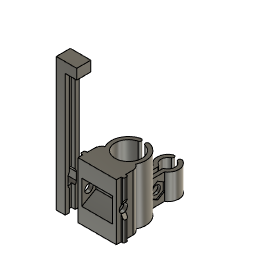
clip (Autodesk Fusion 360 design; units mm, degrees)
Autodesk Fusion 360 part; units mm, degrees
sketch "Sketch1" plane through (0, 0, 0) normal (0, 0, 1) x (1, 0, 0)
  circle A0 centre (0, 0) radius 5.25
  circle A1 centre (0, 0) radius 6.75
  line L0 (0, 1.75) -> (0, 22.5) construction
  line L1 (-7.5, -6.75) -> (7.5, -6.75)
  line L2 (2.25, 11.864) -> (2.25, 6.364)
  line L3 (-2.25, 11.864) -> (-2.25, 6.364)
  circle A2 centre (0, 15.4695) radius 2.75
  circle A3 centre (0, 15.4695) radius 4.25
  line L4 (0.75, 5.1962) -> (0.75, 19.6528)
  line L5 (-0.75, 5.1962) -> (-0.75, 19.6528)
  line L6 (-2, -4.8541) -> (-2, -2)
  arc A4 (2, -2) -> (-2, -2) centre (0, -2) ccw
  line L7 (2, -2) -> (2, -4.8541)
  line L8 (-12.5, -6.75) -> (-12.5, -8.375)
  line L9 (-12.5, -8.375) -> (-14, -8.375)
  line L10 (-14, -8.375) -> (-14, -10.625)
  line L11 (-14, -10.625) -> (-12.5, -10.625)
  line L12 (-12.5, -10.625) -> (-12.5, -12.25)
  line L13 (-16, -12.25) -> (-16, -6.75)
  line L14 (0, -9.5) -> (-16, -9.5) construction
  line L15 (-16, -6.75) -> (-12.5, -6.75)
  line L16 (-16, -12.25) -> (-12.5, -12.25)
  line L17 (-7.5, -6.75) -> (-7.5, -8.625)
  line L18 (-7.5, -8.625) -> (-8.5, -8.625)
  line L19 (-8.5, -8.625) -> (-8.5, -10.375)
  line L20 (-8.5, -10.375) -> (-7.5, -10.375)
  line L21 (-7.5, -10.375) -> (-7.5, -12.25)
  line L22 (-4, -12.25) -> (-4, -6.75)
  line L23 (-7.5, -12.25) -> (7.5, -12.25)
  line L24 (7.5, -12.25) -> (7.5, -10.375)
  line L25 (7.5, -10.375) -> (8.5, -10.375)
  line L26 (8.5, -10.375) -> (8.5, -8.625)
  line L27 (8.5, -8.625) -> (7.5, -8.625)
  line L28 (7.5, -8.625) -> (7.5, -6.75)
  line L29 (4, -6.75) -> (4, -12.25)
  line L30 (-7.5, -6.75) -> (-7.5, -5.75)
  arc A5 (-5.9559, -3.1765) -> (-7.5, -5.75) centre (-4.5833, -5.75) ccw
  line L31 (-4.5833, -5.75) -> (-5.9559, -3.1765) construction
  line L32 (7.5, -6.75) -> (7.5, -5.75)
  arc A6 (7.5, -5.75) -> (5.9559, -3.1765) centre (4.5833, -5.75) ccw
  dimension "d16" = 10.5
  dimension "d17" = 1.5
  dimension "d27" = 1.5
  dimension "d28" = 5.5
  dimension "d29" = 1.5
  dimension "d30" = 1.5
  dimension "d31" = 5.5
  dimension "d32" = 4
  dimension "d65" = 2.25
  dimension "d69" = 1.5
  dimension "d70" = 4
  dimension "d72" = 0.25
  dimension "d73" = 1
  dimension "d74" = 15
  dimension "d79" = 5.5
  dimension "d80" = 5
  dimension "d81" = 2
  dimension "d94" = 1
  constraint coincident A0.centre A1.centre
  constraint concentric A0 A1
  constraint symmetric L1.start L1.end L0
  constraint tangent A1 L1
  constraint coincident A1 L2.end
  constraint parallel L0 L2
  constraint coincident A1 L3.end
  constraint parallel L0 L3
  constraint coincident L0 A2.centre
  constraint concentric A2 A3
  constraint coincident L2.start A3
  constraint coincident L3.start A3
  constraint symmetric L0 L2.end L3.end
  constraint coincident A0 L4.start
  constraint coincident A3 L4.end
  constraint parallel L0 L4
  constraint coincident A0 L5.start
  constraint coincident A3 L5.end
  constraint parallel L0 L5
  constraint symmetric L0 L4.start L5.start
  constraint coincident A0 L6.start
  constraint vertical L6
  constraint tangent L6 A4
  constraint coincident A0 L7.end
  constraint tangent A4 L7
  constraint parallel L6 L7
  constraint symmetric L0 L6.start L7.end
  constraint coincident A0.centre A4
  constraint vertical L8
  constraint perpendicular L8 L9
  constraint perpendicular L9 L10
  constraint perpendicular L10 L11
  constraint perpendicular L11 L12
  constraint horizontal L14
  constraint coincident L0 L14.start
  constraint coincident L13 L14.end
  constraint symmetric L9.end L10.end L14
  constraint coincident L13 L15.start
  constraint coincident L8 L15.end
  constraint perpendicular L8 L15
  constraint coincident L13 L16.start
  constraint coincident L12 L16.end
  constraint perpendicular L12 L16
  constraint symmetric L14 L13.end L13.start
  constraint perpendicular L14 L17
  constraint perpendicular L17 L18
  constraint perpendicular L14 L19
  constraint perpendicular L19 L20
  constraint perpendicular L20 L21
  constraint perpendicular L1 L22
  constraint collinear L17 L21
  constraint symmetric L14 L18.end L19.end
  constraint symmetric L1.start L14 L21.end
  constraint perpendicular L21 L23
  constraint perpendicular L23 L24
  constraint perpendicular L24 L25
  constraint perpendicular L23 L26
  constraint perpendicular L26 L27
  constraint perpendicular L1 L28
  constraint collinear L24 L28
  constraint collinear L18 L27
  constraint collinear L20 L25
  constraint equal L18 L27
  constraint coincident L1 L22.end
  constraint coincident L22.start L23
  constraint coincident L1 L29.start
  constraint coincident L23 L29.end
  constraint perpendicular L23 L29
  constraint symmetric L0 L22.start L29.end
  constraint collinear L16 L23
  constraint collinear L8 L12
  constraint perpendicular L1 L30
  constraint coincident A1 A5.start
  constraint tangent L30 A5
  constraint coincident A5.centre L31.start
  constraint tangent A1 L31
  constraint perpendicular L1 L32
  constraint coincident A1 A6.end
  constraint tangent L32 A6
  constraint symmetric L0 L30.end L32.end
  constraint symmetric L0 A5.start A6.end
  measures "d16" diameter of A0
  measures "d17" distance of A0 A1
  measures "d27" distance of A2 A3
  measures "d28" diameter of A2
  measures "d29" horizontal distance of L2.start L4.end
  measures "d30" distance of L4.end L5.end
  measures "d31" distance of L2.start L2.end
  measures "d32" distance of L6.start L7.end
  measures "d65" distance of L9.end L10.end
  measures "d69" distance of L10.end L11.end
  measures "d70" horizontal distance of L14.start L22.start
  measures "d72" distance of L9 L18
  measures "d73" distance of L19.end L20.end
  measures "d74" distance of L21.end L23.end
  measures "d79" distance of L1.end L23.end
  measures "d80" distance of L1.start L8.start
  measures "d81" distance of L10 L13
  measures "d94" distance of L1.start L30.end
extrude "Extrude3" add sketch "Sketch1" along normal blind 22 contours A0 A1 L4 L5 | A1 L1 L30 A5 | A1 L1 L32 A6 | L1 L22 L23 L29 | L1 L17 L18 L19 L20 L21 L22 L23 | L1 L23 L24 L25 L26 L27 L28 L29 picked at (-2.5299, 5.7021) makes body 1
extrude "Extrude4" add sketch "Sketch1" along normal blind 10 contours A1 L2 A3 L4 | A1 L3 A3 L5 | A2 A3 L4 | A2 A3 L5 bodies 1
extrude "Extrude5" add sketch "Sketch1" along normal blind 2 contours A0 L6 A4 L7 picked at (0, -3.0833) bodies 1
extrude "Extrude6" add sketch "Sketch1" along normal blind 52 separate body contours L8 L9 L10 L11 L12 L13 L15 L16 makes body 2
sketch "Sketch3" plane through (0, 0, 0) normal (1, 0, 0) x (0, 1, 0)
  circle A0 centre (9.114, 5) radius 1.625
  line L0 (6.364, 0) -> (11.864, 0)
  line L1 (11.864, 0) -> (11.864, 10)
  line L2 (11.864, 10) -> (6.364, 10)
  line L3 (9.114, 10) -> (9.114, 0) construction
  line L4 (7.3485, 5) -> (11.864, 5) construction
  line L5 (9.114, 8.1754) -> (6.364, 6.5877)
  line L6 (6.364, 6.5877) -> (6.364, 3.4123)
  line L7 (6.364, 3.4123) -> (9.114, 1.8246)
  line L8 (9.114, 1.8246) -> (11.864, 3.4123)
  line L9 (11.864, 3.4123) -> (11.864, 6.5877)
  line L10 (11.864, 6.5877) -> (9.114, 8.1754)
  circle A1 centre (-9.5, 11) radius 1.625
  line L11 (-9.5, 22) -> (-9.5, 0) construction
  line L12 (-12.25, 0) -> (-12.25, 22)
  line L13 (-6.75, 22) -> (-12.25, 22) construction
  line L14 (-6.75, 0) -> (-12.25, 0) construction
  line L15 (-7.25, 11) -> (-12.25, 11) construction
  line L16 (-6.75, 12.5877) -> (-9.5, 14.1754)
  line L17 (-9.5, 14.1754) -> (-12.25, 12.5877)
  line L18 (-12.25, 12.5877) -> (-12.25, 9.4123)
  line L19 (-12.25, 9.4123) -> (-9.5, 7.8246)
  line L20 (-9.5, 7.8246) -> (-6.75, 9.4123)
  line L21 (-6.75, 9.4123) -> (-6.75, 12.5877)
  line L22 (-9.5, 7.8246) -> (-12.25, 6.2369)
  line L23 (-9.5, 14.1754) -> (-12.25, 15.7631)
  line L24 (6.364, 10) -> (6.364, 0)
  line L25 (-6.75, 0) -> (-6.75, 22) construction
  point P0 (9.114, 5)
  point P1 (-9.5, 11)
  point P2 (-6.75, 0)
  dimension "d49" = 3.25
  dimension "d76" = 3.25
  constraint midpoint L2 L3.start
  constraint midpoint L0 L3.end
  constraint midpoint L1 L4.end
  constraint midpoint P0 L3
  constraint coincident P0 A0.centre
  constraint collinear L1 L9
  constraint vertical L11
  constraint coincident L12.end L13.end
  constraint coincident L12.start L14.end
  constraint midpoint L11.start L13
  constraint midpoint L11.end L14
  constraint midpoint P1 L11
  constraint coincident L12 L15.end
  constraint perpendicular L12 L15
  constraint coincident P1 L15
  constraint coincident P1 A1.centre
  constraint coincident L12 L22.end
  constraint parallel L20 L22
  constraint coincident L12 L23.end
  constraint parallel L16 L23
  constraint coincident P2 L14.start
  constraint perpendicular L13 L25
  constraint collinear L21 L25
  measures "d49" diameter of A0
  measures "d76" diameter of A1
extrude "Extrude7" cut sketch "Sketch3" along normal through all and the other way through all contours A0 | A1 bodies 1
extrude "Extrude8" cut sketch "Sketch3" along normal blind 1 from surface at 1.75 contours L1 L5 L6 L7 L8 L9 L10 L24 bodies 1
extrude "Extrude9" cut sketch "Sketch3" along normal mid plane 12 contours A1 | L12 L19 L22 | L12 L16 L17 L18 L19 L20 L21 | L12 L17 L23 bodies 1
sketch "Sketch4" plane through (0, -12.25, 0) normal (0, -1, 0) x (1, 0, 0)
  line L0 (-6, 6.2369) -> (-6, 15.7631)
  line L1 (-6, 15.7631) -> (6, 15.7631)
  line L2 (6, 15.7631) -> (6, 6.2369)
  line L3 (6, 6.2369) -> (-6, 6.2369)
  line L4 (-7.5, 0) -> (7.5, 0)
  line L5 (7.5, 0) -> (7.5, 22)
  line L6 (7.5, 22) -> (-7.5, 22)
  line L7 (-7.5, 22) -> (-7.5, 0)
  line L8 (-8.5, 0) -> (-8.5, 9.6307) construction
  line L9 (-7.5, 0) -> (-7.5, 22) construction
  line L10 (-7.5, 9.375) -> (-8.5, 7.6429)
  line L11 (-7.5, 9.375) -> (-5.5, 9.375) construction
  line L12 (-8.5, 7.6429) -> (-8.5, 14.3571)
  line L13 (-8.5, 14.3571) -> (-7.5, 12.625)
  line L14 (-7.5, 11) -> (7.5, 11) construction
  line L15 (-7.5, 12.625) -> (-7.5, 9.375)
  line L16 (0, 1.75) -> (0, 22.5)
  line L17 (7.5, 12.625) -> (7.5, 9.375)
  line L18 (8.5, 14.3571) -> (7.5, 12.625)
  line L19 (8.5, 7.6429) -> (8.5, 14.3571)
  line L20 (7.5, 9.375) -> (8.5, 7.6429)
  line L21 (0, 9.375) -> (0, 12.625)
  line L22 (0, 12.625) -> (-7.5, 12.625) construction
  dimension "d84" = 120
  constraint horizontal L11
  constraint coincident L8 L10.end
  constraint parallel L8 L12
  constraint coincident L7 L13.end
  constraint midpoint L9 L14.start
  constraint midpoint L5 L14.end
  constraint symmetric L10.start L13.end L14
  constraint symmetric L10.end L12.end L14
  constraint symmetric L10.start L16 L17.end
  constraint symmetric L10.end L16 L19.start
  constraint symmetric L12.end L16 L18.start
  constraint symmetric L13.end L16 L17.start
  constraint coincident L21.end L22.start
  constraint horizontal L22
  constraint coincident L10.start L11.start
  measures "d84" angle of L10 L11
extrude "Extrude10" cut sketch "Sketch4" along normal through all and the other way through all contours L7 L10 L12 L13 L15 | L5 L17 L18 L19 L20 bodies 1
fillet "Fillet2" radius 0.75 10 edges at (0.75, 12.8238, 5) (-0.75, 12.8238, 5) (0.75, 19.6528, 5) (0.75, 18.1153, 5) (-0.75, 18.1153, 5) (-0.75, 19.6528, 5) (-0.75, 6.7082, 16) (-0.75, 5.1962, 11) (0.75, 6.7082, 16) (0.75, 5.1962, 11) on bodies 1
fillet "Fillet2" radius 0.5 8 edges at (-8.5, -8.625, 18.1785) (-8.5, -10.375, 18.1785) (-8.5, -8.625, 3.8215) (-8.5, -10.375, 3.8215) (8.5, -8.625, 18.1785) (8.5, -10.375, 18.1785) (8.5, -10.375, 3.8215) (8.5, -8.625, 3.8215) on bodies 1
sketch "Sketch6" plane through (-16, 0, 0) normal (-1, 0, 0) x (0, -1, 0)
  line L0 (6.75, 0) -> (12.25, 0)
  line L1 (12.25, 0) -> (12.25, 52)
  line L2 (12.25, 52) -> (6.75, 52)
  line L3 (6.75, 52) -> (6.75, 0)
  line L4 (6.75, 52) -> (12.25, 52)
  line L5 (6.75, 52) -> (6.75, 48)
  line L6 (12.25, 52) -> (12.25, 48)
  line L7 (6.75, 48) -> (12.25, 48)
  circle A0 centre (9.5, 11) radius 1.625 construction
  line L8 (7.875, 12.5) -> (7.875, 9.5)
  arc A1 (7.875, 9.5) -> (11.125, 9.5) centre (9.5, 9.5) ccw
  line L9 (11.125, 9.5) -> (11.125, 12.5)
  arc A2 (11.125, 12.5) -> (7.875, 12.5) centre (9.5, 12.5) ccw
  line L10 (9.5, 11) -> (11.125, 11) construction
  dimension "d96" = 4
  dimension "d99" = 3
  constraint coincident L2.end L3.start
  constraint coincident L3 L5.end
  constraint perpendicular L4 L5
  constraint coincident L1.end L2.start
  constraint coincident L1 L6.end
  constraint perpendicular L4 L6
  constraint perpendicular L6 L7
  constraint vertical L8
  constraint tangent L8 A1
  constraint tangent A1 L9
  constraint parallel L8 L9
  constraint tangent L9 A2
  constraint tangent L8 A2
  constraint tangent A0 L8
  constraint tangent A0 L9
  constraint coincident A0.centre L10.start
  constraint coincident A0 L10.end
  constraint perpendicular L9 L10
  constraint midpoint L9 L10.end
  measures "d96" distance of L1.end L6.end
  measures "d99" distance of A1.end L9.end
extrude "Extrude12" add sketch "Sketch6" against normal blind 8 contours L1 L2 L3 L4 L5 L6 L7 bodies 2
extrude "Extrude13" cut sketch "Sketch6" against normal blind 4 contours L8 A1 L9 A2 bodies 2
